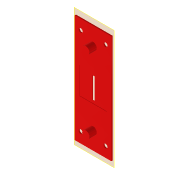
# Autodesk Inventor part: 40_microfluidic_chip_lightsheet_layer1_negative_v0
Saved by Autodesk Inventor 2022 (Build 260153000, 153)
## iProperties
Created: 2021-12-21
Part Number: 40_microfluidic_chip_lightsheet_layer1_negative_v0
Material: Generisch
Document SubType Name: Modeling
Designer: diederichbenedict
Density: 1 g/cm^3
Appearance: Rot
Author: diederichbenedict
Autodesk Inventor part; units mm, degrees
ref_plane "YZ Plane" through (0, 0, 0) normal (1, 0, 0) x (0, 1, 0)
ref_plane "XZ Plane" through (0, 0, 0) normal (0, 1, 0) x (-1, 0, 0)
ref_plane "XY Plane" through (0, 0, 0) normal (0, 0, 1) x (1, 0, 0)
ref_plane "Arbeitsebene1" through (0, 0, 0) normal (0, 0, 1) x (1, 0, 0)
sketch "Skizze1" plane through (0, 0, 0) normal (0, 0, 1) x (1, 0, 0)
  line L0 (-12.5, 37) -> (-12.5, -37) projected
  line L1 (-12.5, -37) -> (12.5, -37) projected
  line L2 (12.5, -37) -> (12.5, 37) projected
  line L3 (12.5, 37) -> (-12.5, 37) projected
  circle A0 centre (8.5, 30) radius 1.4 projected
  circle A1 centre (-8.5, 30) radius 1.4 projected
  circle A2 centre (-8.5, -30) radius 1.4 projected
  circle A3 centre (8.5, -30) radius 1.4 projected
  line L4 (9.25, 9.25) -> (9.25, -9.25) projected
  line L5 (9.25, -9.25) -> (-9.25, -9.25) projected
  line L6 (-9.25, -9.25) -> (-9.25, 9.25) projected
  line L7 (-9.25, 9.25) -> (9.25, 9.25) projected
  arc A4 (0.75, 23.146) -> (-0.75, 23.146) centre (0, 25) ccw projected
  line L8 (0.75, -23.146) -> (0.75, 23.146) projected
  arc A5 (-0.75, -23.146) -> (0.75, -23.146) centre (0, -25) ccw projected
  line L9 (-0.75, 23.146) -> (-0.75, -23.146) projected
  point P0 (0, 0)
extrude "Extrusion1" add sketch "Skizze1" along normal blind 0.4 contours L3 L2 L1 L0 | L4 L5 L8 L7 | L9 L5 L6 L7
sketch "Skizze2" plane through (0, 0, 0.4) normal (0, 0, 1) x (1, 0, 0)
  arc A0 (0.75, 23.146) -> (-0.75, 23.146) centre (0, 25) ccw projected
  line L0 (-12.5, -37) -> (12.5, -37) projected
  line L1 (12.5, -37) -> (12.5, 37) projected
  line L2 (12.5, 37) -> (-12.5, 37) projected
  line L3 (-12.5, 37) -> (-12.5, -37) projected
  circle A1 centre (8.5, -30) radius 1.4 projected
  circle A2 centre (-8.5, -30) radius 1.4 projected
  circle A3 centre (-8.5, 30) radius 1.4 projected
  circle A4 centre (8.5, 30) radius 1.4 projected
  line L4 (0.75, 23.146) -> (0.75, -23.146) projected
  arc A5 (-0.75, -23.146) -> (0.75, -23.146) centre (0, -25) ccw projected
  line L5 (-0.75, -23.146) -> (-0.75, 23.146) projected
  arc A6 (0.75, 23.146) -> (-0.75, 23.146) centre (0, 25) ccw projected
  circle A7 centre (0, 25) radius 2.5
  line L6 (-9.25, 9.25) -> (9.25, 9.25) projected
  line L7 (9.25, -9.25) -> (-9.25, -9.25) projected
  line L8 (0.75, 23.146) -> (0.75, -23.146) projected
  line L9 (0.75, 22.6152) -> (-0.75, 22.6152)
  line L10 (-0.75, 22.6152) -> (-0.75, 9.25)
  line L11 (-0.75, 9.25) -> (0.75, 9.25)
  line L12 (0.75, 9.25) -> (0.75, 22.6152)
  line L13 (-0.75, -23.146) -> (-0.75, 23.146) projected
  line L14 (0.75, -9.25) -> (-0.75, -9.25)
  line L15 (-0.75, -9.25) -> (-0.75, -23.146)
  line L16 (-0.75, -23.146) -> (0.75, -23.146)
  line L17 (0.75, -23.146) -> (0.75, -9.25)
  arc A8 (-0.75, -23.146) -> (0.75, -23.146) centre (0, -25) ccw projected
  circle A9 centre (0, -25) radius 2.5
  line L18 (0.75, 9.25) -> (-0.75, 9.25)
  line L19 (-0.75, 9.25) -> (-0.75, 7.25)
  line L20 (-0.75, 7.25) -> (0.75, 7.25)
  line L21 (0.75, 7.25) -> (0.75, 9.25)
  line L22 (0.75, -9.25) -> (-0.75, -9.25)
  line L23 (-0.75, -9.25) -> (-0.75, -7.25)
  line L24 (-0.75, -7.25) -> (0.75, -7.25)
  line L25 (0.75, -7.25) -> (0.75, -9.25)
  point P0 (0, 0)
  point P1 (0.75, -9.25)
  point P2 (0.75, 9.25)
  point P3 (0.75, -7.25)
  dimension "d2" = 5
  dimension "d11" = 1.5
  dimension "d12" = 2
  dimension "d13" = 2
  constraints: 32 end point, 8 parallel, 6 point on line, 4 horizontal, 4 perpendicular, 2 coincident, 1 centre point, 3 other
  measures "d11" distance of L20.end L19.end
  measures "d12" distance of L19.end L18.end
  measures "d13" distance of L22.end L23.end
extrude "Extrusion2" add sketch "Skizze2" along normal blind 0.4 contours L4 L9 L5 A0 | A0 L5 A7 L4 | L4 L6 L5 A7 | A7 L9 | L4 L20 L5 L6 | L4 L7 L5 L24 | L4 A9 L5 L7 | A9 L5 A5 L4 | L4 L16 L5 A9 | A5 L16 | L3 L2 L1 L0
sketch "Skizze3" plane through (0, 0, 0.8) normal (0, 0, 1) x (1, 0, 0)
  arc A0 (0.75, 23.146) -> (-0.75, 23.146) centre (0, 25) ccw projected
  arc A1 (-0.75, -23.146) -> (0.75, -23.146) centre (0, -25) ccw projected
  arc A2 (0.75, 23.146) -> (-0.75, 23.146) centre (0, 25) ccw projected
  circle A3 centre (0, 25) radius 2.5
  circle A4 centre (0, -25) radius 2.5
  point P0 (0, 0)
  dimension "d5" = 5
  dimension "d6" = 5
  constraints: 2 centre point, 2 coincident
  measures "d5" diameter of A3
  measures "d6" diameter of A4
extrude "Extrusion3" add sketch "Skizze3" along normal blind 5
sketch "Skizze4" plane through (0, 0, 0.8) normal (0, 0, 1) x (1, 0, 0)
  circle A0 centre (0, -25) radius 2.5 projected
  circle A1 centre (0, 25) radius 2.5 projected
  line L0 (12.5, -37) -> (12.5, 37) projected
  line L1 (12.5, 37) -> (-12.5, 37) projected
  line L2 (-12.5, 37) -> (-12.5, -37) projected
  line L3 (-12.5, -37) -> (12.5, -37) projected
  line L4 (-0.75, -7.25) -> (-0.75, 7.25) projected
  line L5 (0.75, 7.25) -> (0.75, -7.25) projected
  circle A2 centre (8.5, -30) radius 1.4 projected
  circle A3 centre (-8.5, -30) radius 1.4 projected
  circle A4 centre (-8.5, 30) radius 1.4 projected
  circle A5 centre (8.5, 30) radius 1.4 projected
  line L6 (-9.25, -9.25) -> (9.25, -9.25)
  line L7 (9.25, -9.25) -> (9.25, 9.25)
  line L8 (9.25, 9.25) -> (-9.25, 9.25)
  line L9 (-9.25, 9.25) -> (-9.25, -9.25)
  line L10 (-9.25, -9.25) -> (9.25, 9.25) construction
  line L11 (9.25, -9.25) -> (-9.25, 9.25) construction
  line L12 (0.75, -7.25) -> (-0.75, -7.25) projected
  line L13 (-0.75, 7.25) -> (0.75, 7.25) projected
  point P0 (0, 0)
  dimension "d9" = 18.5
  dimension "d10" = 18.5
  constraints: 12 end point, 2 midpoint, 2 parallel, 1 horizontal, 1 perpendicular
  measures "d9" distance of L8.end L7.end
  measures "d10" distance of L7.end L6.end
extrude "Extrusion4" cut sketch "Skizze4" against normal blind 0.3 contours L9 L8 L7 L6
equation "\"d7\" = d6"
